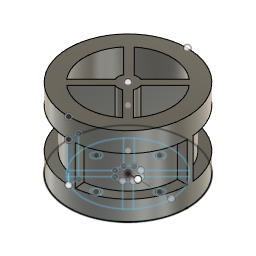
Driving_wheel v1 (Autodesk Fusion 360 design; units mm, degrees)
Autodesk Fusion 360 part; units mm, degrees
sketch "Sketch1" plane through (0, 0, 0) normal (0, 0, 1) x (1, 0, 0) in component "Wheel"
  circle A0 centre (0, 0) radius 15
  circle A1 centre (-0.0001, 8) radius 1.125
  circle A2 centre (-8, 0) radius 1.125
  circle A3 centre (-0.0473, -7.9999) radius 1.125
  circle A4 centre (8, 0.0001) radius 1.125
  circle A5 centre (0, 0) radius 11
  circle A6 centre (0, 0) radius 2.5
  line L0 (0, 0) -> (11, 0) construction
  line L1 (0, 0) -> (2.5, 0) construction
  line L2 (0, 0) -> (2.5, 0) construction
  line L3 (2.3097, 0.9567) -> (8.4252, 7.0722)
  line L4 (0.9567, 2.3097) -> (7.0722, 8.4252)
  line L5 (0, 0) -> (2.5, 0) construction
  line L6 (0, 0) -> (2.5, 0) construction
  line L7 (0, 0) -> (2.5, 0) construction
  line L8 (0, 0) -> (2.5, 0) construction
  line L9 (-2.3097, -0.9567) -> (-8.4252, -7.0722)
  line L10 (-0.9567, -2.3097) -> (-7.0722, -8.4252)
  line L11 (-2.232, 1.126) -> (-8.3115, 7.2055)
  line L12 (-0.7821, 2.3745) -> (-6.9411, 8.5335)
  line L13 (0, 0) -> (2.5, 0) construction
  line L14 (0, 0) -> (2.5, 0) construction
  line L15 (0, 0) -> (2.5, 0) construction
  line L16 (0.9567, -2.3097) -> (7.0722, -8.4252)
  line L17 (2.3097, -0.9567) -> (8.4252, -7.0722)
  point P0 (-0.0001, 8)
  point P1 (-0.0473, -7.9999)
  point P2 (8, 0.0001)
  point P3 (-8, 0)
  point P4 (-2.3097, -0.9567)
  point P5 (-0.9567, -2.3097)
  point P6 (-2.232, 1.126)
  point P7 (-0.7821, 2.3745)
  dimension "d1" = 30
  dimension "d3" = 2.25
  dimension "d4" = 2.25
  dimension "d5" = 2.25
  dimension "d6" = 2.25
  dimension "d7" = 22
  dimension "d8" = 5
  constraint coincident A0.centre A5.centre
  constraint coincident P0 A1.centre
  constraint coincident P3 A2.centre
  constraint coincident P1 A3.centre
  constraint coincident P2 A4.centre
  constraint concentric A5 A6
  constraint horizontal L0
  constraint horizontal L1
  constraint horizontal L2
  constraint coincident A5 L3.end
  constraint coincident A5 L4.end
  constraint parallel L3 L4
  constraint horizontal L5
  constraint horizontal L6
  constraint horizontal L7
  constraint horizontal L8
  constraint coincident A5 L9.end
  constraint coincident A5 L10.end
  constraint coincident P4 L9.start
  constraint coincident P5 L10.start
  constraint coincident A6 P6
  constraint coincident A6 P7
  constraint coincident P6 L11.start
  constraint coincident A5 L11.end
  constraint coincident P7 L12.start
  constraint coincident A5 L12.end
  constraint horizontal L13
  constraint horizontal L14
  constraint horizontal L15
  constraint coincident A5 L16.end
  constraint coincident A5 L17.end
  constraint parallel L16 L17
  measures "d1" diameter of A0
  measures "d3" diameter of A1
  measures "d4" diameter of A2
  measures "d5" diameter of A3
  measures "d6" diameter of A4
  measures "d7" diameter of A5
  measures "d8" diameter of A6
extrude "Extrude1" add sketch "Sketch1" along normal blind 20 contours A0 | A5 A6 L3 L4 | A5 A6 L16 L17 | A6 | A5 A6 L11 L12 | A5 A6 L9 L10 makes body 1 in component "Wheel"
extrude "Extrude2" add sketch "Sketch1" along normal blind 4 contours A5 A6 L3 L17 | A5 A6 L4 L12 | A5 A6 L10 L16 | A5 A6 L9 L11 bodies 1 in component "Wheel"
sketch "Sketch2" plane through (0, 0, 0) normal (1, 0, 0) x (0, 1, 0) in component "Wheel"
  line L0 (-15, 15) -> (-12.5, 15)
  line L1 (-12.5, 15) -> (-12.5, 5)
  line L2 (-12.5, 5) -> (-15, 5)
  line L3 (-15, 5) -> (-15, 15)
  point P0 (0, 20)
  point P1 (15, 20)
  point P2 (-15, 20)
  point P3 (0, 15)
  point P4 (0, 5)
  point P5 (-15, 5)
  point P6 (-15, 15)
  point P7 (-15, 15)
  point P8 (-12.5, 15)
  point P9 (-12.5, 5)
  constraint coincident P7 P6
  constraint coincident P8 L0.end
  constraint coincident P9 L1.end
  constraint perpendicular L0 L1
  constraint perpendicular L1 L2
  constraint coincident P6 L0.start
  constraint perpendicular L2 L3
revolve "Revolve1" cut sketch "Sketch2" angle 360 about axis through (0, 0, 0) along (0, 0, -1) bodies 1 in component "Wheel"
revolve "Revolve2" add sketch "Sketch2" angle 6 about axis through (0, 0, 15) along (0, 0, 1) separate body makes body 2 in component "Wheel"
pattern_circular "C-Pattern1" count 4 over 360 about axis through (0, 0, 5) along (0, 0, 1) of bodies 2 makes body 3 at (14.1667, 0, 11.6667) makes body 4 at (0, 14.1667, 11.6667) makes body 5 at (-14.1667, 0, 11.6667) in component "Wheel"
combine "Combine1" operation add target body 1 tool bodies 5 2 3 4 in component "Wheel"
sketch "Sketch3" plane through (0, 0, 0) normal (0, 1, 0) x (1, 0, 0) in component "Wheel"
component "Wheel" placed x (1, 0, 0) y (0, 1, 0) z (0, 0, 1) at (0, 0, 0)
